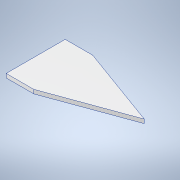
# Autodesk Inventor part: Wedge_base
Saved by Autodesk Inventor 2020 (Build 240168000, 168)
## iProperties
Created: 2020-01-30
Part Number: Wedge_base
Material: Aluminum 6061
Document SubType Name: Modeling
Designer: Connor
Density: 2.7 g/cm^3
Appearance: Aluminum - Flat
Mass: 701.162 g
Surface Area: 592.255 cm^2
Volume: 259.69 cm^3
Author: Connor
Autodesk Inventor part; units mm, degrees
ref_plane "YZ Plane" through (0, 0, 0) normal (1, 0, 0) x (0, 1, 0)
ref_plane "XZ Plane" through (0, 0, 0) normal (0, 1, 0) x (-1, 0, 0)
ref_plane "XY Plane" through (0, 0, 0) normal (0, 0, 1) x (1, 0, 0)
sketch "Sketch1" plane through (0, 0, 0) normal (0, 1, 0) x (-1, 0, 0)
  line L0 (0, 0) -> (0, -150)
  line L1 (0, 0) -> (-70.096, 0)
  line L2 (-70.096, 0) -> (-276.1568, -75)
  line L3 (0, -150) -> (-70.096, -150)
  line L4 (-70.096, -150) -> (-276.1568, -75)
  dimension "d0" = 150
  dimension "d1" = 70.096
  dimension "d2" = 160
  dimension "d3" = 160
  constraints: 10 end point, 2 horizontal, 1 parallel, 1 vertical
  measures "d0" distance of L0.start L0.end
  measures "d1" distance of L0.start L1.end
  measures "d2" angle of L2 L1
  measures "d3" angle of L4 L3
extrude "Extrusion1" add sketch "Sketch1" along normal blind 10
equation "\"d3\" = d2"
body "Solid1"
